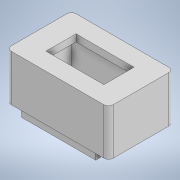
# Autodesk Inventor part: Black_Keyboard_Button_Base
Saved by Autodesk Inventor 2021 (Build 250183000, 183)
## iProperties
Created: 2020-06-05
Part Number: Black_Keyboard_Button_Base
Material: Generic
Document SubType Name: Modeling
Designer: ameli
Density: 1 g/cm^3
Appearance: Default
Author: ameli
Autodesk Inventor part; units mm, degrees
ref_plane "YZ Plane" through (0, 0, 0) normal (1, 0, 0) x (0, 1, 0)
ref_plane "XZ Plane" through (0, 0, 0) normal (0, 1, 0) x (-1, 0, 0)
ref_plane "XY Plane" through (0, 0, 0) normal (0, 0, 1) x (1, 0, 0)
sketch "Sketch1" plane through (0, 0, 0) normal (0, 1, 0) x (-1, 0, 0)
  line L0 (11, 7) -> (-11, 7)
  line L1 (-11, 7) -> (-11, -7)
  line L2 (-11, -7) -> (11, -7)
  line L3 (11, -7) -> (11, 7)
  point P0 (0, 0)
  dimension "d0" = 22
  dimension "d1" = 14
  dimension "d2" = 7
  dimension "d3" = 11
  constraints: 8 end point, 2 parallel, 1 horizontal, 1 perpendicular
  measures "d0" distance of L1.end L2.end
  measures "d1" distance of L2.end L0.start
  measures "d2" distance from line of L0 point (0, 0)
  measures "d3" distance from line of point (0, 0) L3
extrude "Extrusion1" add sketch "Sketch1" along normal blind 10
fillet "Fillet1" radius 1 4 edges at (11, 5, 7) (11, 5, -7) (-11, 5, -7) (-11, 5, 7)
shell "Shell1" thickness 1.5 removed faces 1 at (-3.3333, 0, -2.3333)
sketch "Sketch2" plane through (0, 10, 0) normal (0, 1, 0) x (1, 0, 0)
  line L0 (-6.25, 3.25) -> (6.25, 3.25)
  line L1 (6.25, 3.25) -> (6.25, -3.25)
  line L2 (6.25, -3.25) -> (-6.25, -3.25)
  line L3 (-6.25, -3.25) -> (-6.25, 3.25)
  point P0 (0, 0)
  dimension "d8" = 6.5
  dimension "d9" = 12.5
  dimension "d10" = 3.25
  dimension "d11" = 6.25
  constraints: 8 end point, 2 parallel, 1 horizontal, 1 perpendicular
  measures "d8" distance of L0.end L1.end
  measures "d9" distance of L0.start L0.end
  measures "d10" distance from line of point (0, 0) L0
  measures "d11" distance from line of point (0, 0) L1
extrude "Extrusion2" cut sketch "Sketch2" against normal blind 10
sketch "Sketch4" plane through (0, 0, 0) normal (0, -1, 0) x (1, 0, 0)
  line L0 (8, 6.75) -> (-8, 6.75)
  line L1 (-8, 6.75) -> (-8, 5.75)
  line L2 (-8, 5.75) -> (8, 5.75)
  line L3 (8, 5.75) -> (8, 6.75)
  line L4 (11, 6) -> (11, -6) projected
  line L5 (-9.5, 5.5) -> (9.5, 5.5) projected
  line L6 (8, -5.75) -> (-8, -5.75)
  line L7 (-8, -5.75) -> (-8, -6.75)
  line L8 (-8, -6.75) -> (8, -6.75)
  line L9 (8, -6.75) -> (8, -5.75)
  line L10 (-11, -6) -> (-11, 6) projected
  line L11 (9.5, -5.5) -> (-9.5, -5.5) projected
  point P0 (0, 0)
  dimension "d19" = 1
  dimension "d20" = 16
  dimension "d21" = 3
  dimension "d22" = 0.25
  dimension "d23" = 16
  dimension "d24" = 1
  dimension "d25" = 3
  dimension "d26" = 0.25
  constraints: 16 end point, 4 parallel, 2 horizontal, 2 perpendicular
  measures "d19" distance of L0.end L1.end
  measures "d20" distance of L0.start L0.end
  measures "d21" distance between parallel lines of L4 L3
  measures "d22" distance between parallel lines of L5 L2
  measures "d23" distance of L7.end L8.end
  measures "d24" distance of L8.end L6.start
  measures "d25" distance between parallel lines of L10 L7
  measures "d26" distance between parallel lines of L11 L6
extrude "Extrusion3" add sketch "Sketch4" along normal blind 1.5
body "Solid1"
